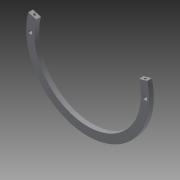
# Autodesk Inventor part: TopfemaleHoopSection_v1
Saved by Autodesk Inventor 2013 (Build 170138000, 138)
## iProperties
Created: 2013-01-17
Part Number: TopfemaleHoopSection_v1
Material: Generic
Document SubType Name: Modeling
Designer: twsass
Density: 1 g/cm^3
Author: twsass
Autodesk Inventor part; units mm, degrees
ref_plane "YZ Plane" through (0, 0, 0) normal (1, 0, 0) x (0, 1, 0)
ref_plane "XZ Plane" through (0, 0, 0) normal (0, 1, 0) x (-1, 0, 0)
ref_plane "XY Plane" through (0, 0, 0) normal (0, 0, 1) x (1, 0, 0)
sketch "Sketch1" plane through (0, 0, 0) normal (0, 0, 1) x (1, 0, 0)
  circle A0 centre (162.4314, 6.464) radius 168.91
  circle A1 centre (162.4314, 6.464) radius 146.05
  line L0 (162.4314, 6.464) -> (325.586, 50.1811)
  line L1 (162.4314, 6.464) -> (331.3414, 6.464) construction
  line L2 (162.4314, 6.464) -> (-0.7231, 50.1811)
  line L3 (162.4314, 6.464) -> (331.3414, 6.464) construction
  line L4 (21.358, 44.2645) -> (-0.7231, 50.1811)
  line L5 (325.586, 50.1811) -> (303.5049, 44.2645)
  point P0 (0, 0)
  point P1 (308.4814, 6.464)
  point P2 (16.3814, 6.464)
  dimension "d18" = 337.82
  dimension "d20" = 292.1
  dimension "d21" = 15
  dimension "d22" = 165
  dimension "d23" = 162.56
  constraints: 12 end point, 6 point on circle, 2 centre point, 2 equal length, 2 horizontal, 2 point on line, 1 coincident, 1 collinear
  measures "d18" diameter of A0
  measures "d20" diameter of A1
  measures "d21" angle of L1 L0
  measures "d22" angle of L3 L2
  measures "d23" distance of A0.centre point (0, 0)
extrude "Extrusion6" add sketch "Sketch1" along normal blind 12.7 contours A0 L2 A1 L0 picked at (5.3976, 42.3533)
sketch "Sketch5" plane through (-0.7231, 50.1811, 12.7) normal (0.258819, 0.9659258, 0) x (0.9659258, -0.258819, 0)
  line L0 (22.86, 12.7) -> (0, 12.7) projected
  line L1 (22.86, 12.7) -> (22.86, 0) projected
  circle A0 centre (11.43, 6.35) radius 3.175
  point P0 (13.6863, 12.7)
  dimension "d26" = 6.35
  dimension "d27" = 6.35
  dimension "d28" = 11.43
  constraints: 1 centre point
  measures "d26" diameter of A0
  measures "d27" distance from line of L0 A0.centre
  measures "d28" distance from line of L1 A0.centre
extrude "Extrusion7" cut sketch "Sketch5" against normal blind 12.7
sketch "Sketch6" plane through (303.5049, 44.2645, 12.7) normal (-0.258819, 0.9659258, 0) x (0.9659258, 0.258819, 0)
  line L0 (22.86, 12.7) -> (0, 12.7) projected
  line L1 (0, 12.7) -> (0, 0) projected
  circle A0 centre (11.43, 6.35) radius 3.175
  point P0 (-304.6197, 12.7)
  dimension "d31" = 6.35
  dimension "d32" = 6.35
  dimension "d33" = 11.43
  constraints: 1 centre point
  measures "d31" diameter of A0
  measures "d32" distance from line of L0 A0.centre
  measures "d33" distance from line of L1 A0.centre
extrude "Extrusion8" cut sketch "Sketch6" against normal blind 12.7
sketch "Sketch7" plane through (0, 0, 12.7) normal (0, 0, 1) x (1, 0, 0)
  arc A0 (-0.7231, 50.1811) -> (325.586, 50.1811) centre (162.4314, 6.464) ccw projected
  line L0 (162.4314, 6.464) -> (4.9514, 6.464)
  line L1 (4.9514, 6.464) -> (10.0314, 6.464)
  line L2 (10.0314, 6.464) -> (10.0314, 1.7015)
  line L3 (10.0314, 1.7015) -> (-0.1286, 1.7015)
  line L4 (-0.1286, 1.7015) -> (-0.1286, 11.2265)
  line L5 (-0.1286, 11.2265) -> (10.0314, 11.2265)
  line L6 (10.0314, 11.2265) -> (10.0314, 6.464)
  point P0 (0, 0)
  dimension "d36" = 157.48
  dimension "d38" = 5.08
  dimension "d39" = 4.7625
  dimension "d40" = 10.16
  dimension "d41" = 9.525
  constraints: 14 end point, 3 perpendicular, 2 parallel, 1 horizontal, 1 point on line, 1 other
  measures "d36" distance of L0.start L0.end
  measures "d38" distance of L0.end L1.end
  measures "d39" distance of L1.end L2.end
  measures "d40" distance of L2.end L3.end
  measures "d41" distance of L3.end L4.end
extrude "Extrusion9" cut sketch "Sketch7" against normal blind 25.4
sketch "Sketch8" plane through (0, 0, 12.7) normal (0, 0, 1) x (1, 0, 0)
  line L0 (-0.1286, 1.7015) -> (-0.1286, 11.2265) projected
  arc A0 (-0.7231, 50.1811) -> (325.586, 50.1811) centre (162.4314, 6.464) ccw projected
  line L1 (162.4314, 6.464) -> (319.9114, 6.464)
  line L2 (319.9114, 6.464) -> (319.9114, 11.2265)
  line L3 (319.9114, 11.2265) -> (324.9914, 11.2265)
  line L4 (324.9914, 11.2265) -> (324.9914, 1.7015)
  line L5 (324.9914, 1.7015) -> (314.8314, 1.7015)
  line L6 (314.8314, 1.7015) -> (314.8314, 11.2265)
  line L7 (314.8314, 11.2265) -> (324.9914, 11.2265)
  point P0 (0, 0)
  dimension "d44" = 157.48
  dimension "d45" = 4.7625
  dimension "d46" = 5.08
  dimension "d47" = 9.525
  dimension "d48" = 10.16
  constraints: 14 end point, 3 parallel, 3 perpendicular, 1 collinear, 1 other
  measures "d44" distance of L1.start L1.end
  measures "d45" distance of L1.end L2.end
  measures "d46" distance of L2.end L3.end
  measures "d47" distance of L3.end L4.end
  measures "d48" distance of L4.end L5.end
extrude "Extrusion10" cut sketch "Sketch8" against normal blind 25.4
body "Solid3"
